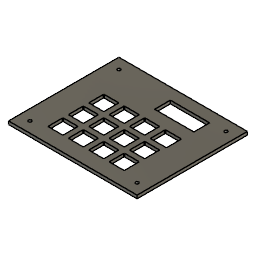
plate (Autodesk Fusion 360 design; units mm, degrees)
part number: 2026-02-28-20-48-28-923
Autodesk Fusion 360 part; units mm, degrees
sketch "plate-2026-02-28T17_07_32.054Z" plane through (0, 0, 0) normal (0, 0, 1) x (1, 0, 0)
  line L0 (3.025, 52.475) -> (16.025, 52.475)
  line L1 (3.025, 38.475) -> (16.025, 38.475)
  line L2 (2.525, 51.975) -> (2.525, 38.975)
  line L3 (16.525, 51.975) -> (16.525, 38.975)
  arc A0 (3.025, 52.475) -> (2.525, 51.975) centre (3.025, 51.975) ccw
  arc A1 (16.525, 51.975) -> (16.025, 52.475) centre (16.025, 51.975) ccw
  arc A2 (2.525, 38.975) -> (3.025, 38.475) centre (3.025, 38.975) ccw
  arc A3 (16.025, 38.475) -> (16.525, 38.975) centre (16.025, 38.975) ccw
  line L4 (22.075, 52.475) -> (35.075, 52.475)
  line L5 (22.075, 38.475) -> (35.075, 38.475)
  line L6 (21.575, 51.975) -> (21.575, 38.975)
  line L7 (35.575, 51.975) -> (35.575, 38.975)
  arc A4 (22.075, 52.475) -> (21.575, 51.975) centre (22.075, 51.975) ccw
  arc A5 (35.575, 51.975) -> (35.075, 52.475) centre (35.075, 51.975) ccw
  arc A6 (21.575, 38.975) -> (22.075, 38.475) centre (22.075, 38.975) ccw
  arc A7 (35.075, 38.475) -> (35.575, 38.975) centre (35.075, 38.975) ccw
  line L8 (41.125, 52.475) -> (54.125, 52.475)
  line L9 (41.125, 38.475) -> (54.125, 38.475)
  line L10 (40.625, 51.975) -> (40.625, 38.975)
  line L11 (54.625, 51.975) -> (54.625, 38.975)
  arc A8 (41.125, 52.475) -> (40.625, 51.975) centre (41.125, 51.975) ccw
  arc A9 (54.625, 51.975) -> (54.125, 52.475) centre (54.125, 51.975) ccw
  arc A10 (40.625, 38.975) -> (41.125, 38.475) centre (41.125, 38.975) ccw
  arc A11 (54.125, 38.475) -> (54.625, 38.975) centre (54.125, 38.975) ccw
  line L12 (60.3652, 52.475) -> (74.4538, 52.475)
  line L13 (60.4135, 38.475) -> (74.4538, 38.475)
  line L14 (59.9891, 51.6556) -> (59.9891, 38.7106)
  line L15 (74.9538, 51.975) -> (74.9538, 38.975)
  arc A12 (60.3652, 52.475) -> (59.9891, 51.6556) centre (60.3737, 51.9751) ccw
  arc A13 (74.9538, 51.975) -> (74.4538, 52.475) centre (74.4538, 51.975) ccw
  arc A14 (59.9891, 38.7106) -> (60.4135, 38.475) centre (60.4135, 38.975) ccw
  arc A15 (74.4538, 38.475) -> (74.9538, 38.975) centre (74.4538, 38.975) ccw
  line L16 (3.025, 33.425) -> (16.025, 33.425)
  line L17 (3.025, 19.425) -> (16.025, 19.425)
  line L18 (2.525, 32.925) -> (2.525, 19.925)
  line L19 (16.525, 32.925) -> (16.525, 19.925)
  arc A16 (3.025, 33.425) -> (2.525, 32.925) centre (3.025, 32.925) ccw
  arc A17 (16.525, 32.925) -> (16.025, 33.425) centre (16.025, 32.925) ccw
  arc A18 (2.525, 19.925) -> (3.025, 19.425) centre (3.025, 19.925) ccw
  arc A19 (16.025, 19.425) -> (16.525, 19.925) centre (16.025, 19.925) ccw
  line L20 (22.075, 33.425) -> (35.075, 33.425)
  line L21 (22.075, 19.425) -> (35.075, 19.425)
  line L22 (21.575, 32.925) -> (21.575, 19.925)
  line L23 (35.575, 32.925) -> (35.575, 19.925)
  arc A20 (22.075, 33.425) -> (21.575, 32.925) centre (22.075, 32.925) ccw
  arc A21 (35.575, 32.925) -> (35.075, 33.425) centre (35.075, 32.925) ccw
  arc A22 (21.575, 19.925) -> (22.075, 19.425) centre (22.075, 19.925) ccw
  arc A23 (35.075, 19.425) -> (35.575, 19.925) centre (35.075, 19.925) ccw
  line L24 (41.125, 33.425) -> (54.125, 33.425)
  line L25 (41.125, 19.425) -> (54.125, 19.425)
  line L26 (40.625, 32.925) -> (40.625, 19.925)
  line L27 (54.625, 32.925) -> (54.625, 19.925)
  arc A24 (41.125, 33.425) -> (40.625, 32.925) centre (41.125, 32.925) ccw
  arc A25 (54.625, 32.925) -> (54.125, 33.425) centre (54.125, 32.925) ccw
  arc A26 (40.625, 19.925) -> (41.125, 19.425) centre (41.125, 19.925) ccw
  arc A27 (54.125, 19.425) -> (54.625, 19.925) centre (54.125, 19.925) ccw
  line L28 (60.175, 33.425) -> (73.175, 33.425)
  line L29 (60.175, 19.425) -> (73.175, 19.425)
  line L30 (59.675, 32.925) -> (59.675, 19.925)
  line L31 (73.675, 32.925) -> (73.675, 19.925)
  arc A28 (60.175, 33.425) -> (59.675, 32.925) centre (60.175, 32.925) ccw
  arc A29 (73.675, 32.925) -> (73.175, 33.425) centre (73.175, 32.925) ccw
  arc A30 (59.675, 19.925) -> (60.175, 19.425) centre (60.175, 19.925) ccw
  arc A31 (73.175, 19.425) -> (73.675, 19.925) centre (73.175, 19.925) ccw
  line L32 (3.025, 14.375) -> (16.025, 14.375)
  line L33 (3.025, 0.375) -> (16.025, 0.375)
  line L34 (2.525, 13.875) -> (2.525, 0.875)
  line L35 (16.525, 13.875) -> (16.525, 0.875)
  arc A32 (3.025, 14.375) -> (2.525, 13.875) centre (3.025, 13.875) ccw
  arc A33 (16.525, 13.875) -> (16.025, 14.375) centre (16.025, 13.875) ccw
  arc A34 (2.525, 0.875) -> (3.025, 0.375) centre (3.025, 0.875) ccw
  arc A35 (16.025, 0.375) -> (16.525, 0.875) centre (16.025, 0.875) ccw
  line L36 (22.075, 14.375) -> (35.075, 14.375)
  line L37 (22.075, 0.375) -> (35.075, 0.375)
  line L38 (21.575, 13.875) -> (21.575, 0.875)
  line L39 (35.575, 13.875) -> (35.575, 0.875)
  arc A36 (22.075, 14.375) -> (21.575, 13.875) centre (22.075, 13.875) ccw
  arc A37 (35.575, 13.875) -> (35.075, 14.375) centre (35.075, 13.875) ccw
  arc A38 (21.575, 0.875) -> (22.075, 0.375) centre (22.075, 0.875) ccw
  arc A39 (35.075, 0.375) -> (35.575, 0.875) centre (35.075, 0.875) ccw
  line L40 (41.125, 14.375) -> (54.125, 14.375)
  line L41 (41.125, 0.375) -> (54.125, 0.375)
  line L42 (40.625, 13.875) -> (40.625, 0.875)
  line L43 (54.625, 13.875) -> (54.625, 0.875)
  arc A40 (41.125, 14.375) -> (40.625, 13.875) centre (41.125, 13.875) ccw
  arc A41 (54.625, 13.875) -> (54.125, 14.375) centre (54.125, 13.875) ccw
  arc A42 (40.625, 0.875) -> (41.125, 0.375) centre (41.125, 0.875) ccw
  arc A43 (54.125, 0.375) -> (54.625, 0.875) centre (54.125, 0.875) ccw
  line L44 (60.175, 14.375) -> (73.175, 14.375)
  line L45 (60.175, 0.375) -> (73.175, 0.375)
  line L46 (59.675, 13.875) -> (59.675, 0.875)
  line L47 (73.675, 13.875) -> (73.675, 0.875)
  arc A44 (60.175, 14.375) -> (59.675, 13.875) centre (60.175, 13.875) ccw
  arc A45 (73.675, 13.875) -> (73.175, 14.375) centre (73.175, 13.875) ccw
  arc A46 (59.675, 0.875) -> (60.175, 0.375) centre (60.175, 0.875) ccw
  arc A47 (73.175, 0.375) -> (73.675, 0.875) centre (73.175, 0.875) ccw
  line L48 (-20.37, -13.56) -> (99.63, -13.56)
  line L49 (-20.3699, 89.4901) -> (99.63, 89.49)
  line L50 (-20.37, -13.56) -> (-20.3699, 89.4901)
  line L51 (99.63, -13.56) -> (99.63, 89.49)
  line L52 (38.4188, 78.6901) -> (75, 78.6901)
  line L53 (75, 78.6901) -> (75, 64.0864)
  line L54 (75, 64.0864) -> (38.4188, 64.0864)
  line L55 (38.4188, 64.0864) -> (38.4188, 78.6901)
  circle A48 centre (-10.3699, 79.4901) radius 1.45
  circle A49 centre (89.63, 79.49) radius 1.45
  circle A50 centre (89.63, -3.56) radius 1.45
  circle A51 centre (-10.37, -3.56) radius 1.45
  dimension "d15" = 2.9
  dimension "d16" = 2.9
  dimension "d17" = 2.9
  dimension "d18" = 2.9
  dimension "d19" = 10
  dimension "d20" = 10
  dimension "d21" = 10
  dimension "d22" = 10
  dimension "d23" = 10
  dimension "d24" = 10
  dimension "d25" = 10
  dimension "d26" = 10
  constraint horizontal L52
  constraint vertical L53
  constraint horizontal L54
  constraint vertical L55
  measures "d15" diameter of A48
  measures "d16" diameter of A49
  measures "d17" diameter of A50
  measures "d18" diameter of A51
  measures "d19" distance of L48 A51.centre
  measures "d20" distance of L50 A51.centre
  measures "d21" distance of L48 A50.centre
  measures "d22" distance of L51 A50.centre
  measures "d23" distance of L49 A49.centre
  measures "d24" distance of L51 A49.centre
  measures "d25" distance of L49 A48.centre
  measures "d26" distance of L50 A48.centre
extrude "Extrude2" add sketch "plate-2026-02-28T17_07_32.054Z" along normal blind 3
